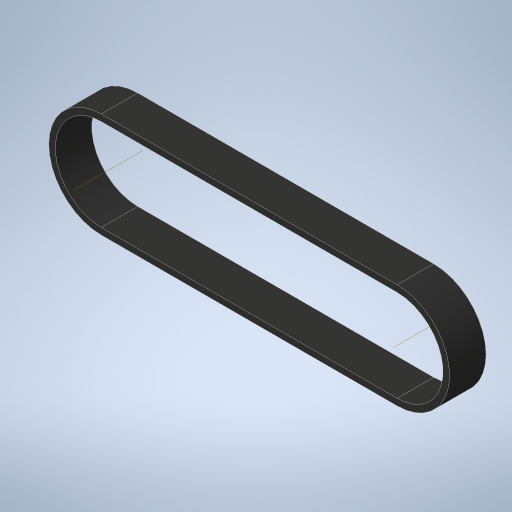
# Autodesk Inventor part: BELT
Saved by Autodesk Inventor 2023.3 (Build 273359000, 359)
## iProperties
RuleStatus: InUse
Created: 2019-01-18
Part Number: BELT
Material: Rubber
Document SubType Name: Modeling
Designer: pctech
Density: 0.93 g/cm^3
Appearance: Rubber - Black
AfterDocOpen0: show
AfterDocNew0: show
Author: pctech
Autodesk Inventor part; units mm, degrees
ref_plane "YZ Plane" through (0, 0, 0) normal (1, 0, 0) x (0, 1, 0)
ref_plane "XZ Plane" through (0, 0, 0) normal (0, 1, 0) x (-1, 0, 0)
ref_plane "XY Plane" through (0, 0, 0) normal (0, 0, 1) x (1, 0, 0)
sketch "Sketch1" plane through (0, 0, 0) normal (0, 0, 1) x (1, 0, 0)
  arc A0 (0, -11.4595) -> (0, 11.4595) centre (0, 0) ccw construction
  arc A1 (-68.9989, 11.4595) -> (-68.9989, -11.4595) centre (-68.9989, 0) ccw construction
  line L0 (0, -11.4595) -> (-68.9989, -11.4595) construction
  line L1 (0, 11.4595) -> (-68.9989, 11.4595) construction
  dimension "Belt_Teeth" = 70
  dimension "Belt_Pitch2" = 3
  dimension "d0" = 22.919
  dimension "d1" = 22.919
  dimension "d2" = 36.0011
  dimension "d3" = 36.0011
  dimension "Center_Distance" = 68.9989
  dimension "d5" = 68.9989
  constraints: 4 end point, 4 point on circle, 4 tangent, 2 centre point, 1 coincident, 1 horizontal alignment
  measures "d0" diameter of A0
  measures "d1" diameter of A1
  measures "Center_Distance" distance of A1.centre point (0, 0)
  measures "d5" distance of L1.start L1.end
sketch "Sketch2" plane through (0, 0, 0) normal (0, 0, 1) x (1, 0, 0)
  line L0 (35.7235, 34.2567) -> (38.7235, 34.2567)
  point P0 (0, 0)
  dimension "Belt_Pitch2" = 3
  constraints: 2 end point, 1 horizontal
  measures "Belt_Pitch2" distance of L0.start L0.end
sketch "Sketch4" plane through (0, 0, 0) normal (0, 0, 1) x (1, 0, 0)
  line L0 (-16.1422, -21.869) -> (-14.1422, -21.869)
  line L1 (-16.1422, -21.869) -> (-16.1422, -20.349)
  arc A0 (-15.5872, -20.904) -> (-16.1422, -20.349) centre (-16.1422, -20.904) ccw
  line L2 (-15.5872, -20.904) -> (-15.5872, -20.959)
  arc A1 (-15.5872, -20.959) -> (-15.4372, -21.109) centre (-15.4372, -20.959) ccw
  line L3 (-15.4372, -21.109) -> (-14.8472, -21.109)
  line L4 (-14.1422, -21.869) -> (-14.1422, -20.349)
  arc A2 (-14.1422, -20.349) -> (-14.6972, -20.904) centre (-14.1422, -20.904) ccw
  arc A3 (-14.8472, -21.109) -> (-14.6972, -20.959) centre (-14.8472, -20.959) ccw
  line L5 (-14.6972, -20.959) -> (-14.6972, -20.904)
  line L6 (0, 11.4595) -> (-68.9989, 11.4595) construction
  arc A4 (-68.9989, 11.4595) -> (-68.9989, -11.4595) centre (-68.9989, 0) ccw construction
  line L7 (0, -11.4595) -> (-68.9989, -11.4595) construction
  arc A5 (0, -11.4595) -> (0, 11.4595) centre (0, 0) ccw construction
  arc A6 (-68.9989, 12.2195) -> (-68.9989, -12.2195) centre (-68.9989, 0) ccw
  line L8 (-68.9989, 12.2195) -> (0, 12.2195)
  arc A7 (0, -12.2195) -> (0, 12.2195) centre (0, 0) ccw
  line L9 (0, -12.2195) -> (-68.9989, -12.2195)
  arc A8 (-68.9989, 10.6995) -> (-68.9989, -10.6995) centre (-68.9989, 0) ccw
  line L10 (-68.9989, 10.6995) -> (0, 10.6995)
  arc A9 (0, -10.6995) -> (0, 10.6995) centre (0, 0) ccw
  line L11 (0, -10.6995) -> (-68.9989, -10.6995)
  point P0 (-15.1422, -21.109)
  point P1 (-15.1422, -21.869)
  dimension "d9" = 2
  dimension "d10" = 1.52
  dimension "d11" = 0.76
  dimension "d12" = 0.555
  dimension "d13" = 0.555
  dimension "d14" = 0.15
  dimension "d15" = 0.15
  dimension "belt_thickness" = 1.52
  dimension "d44" = 0.76
  constraints: 20 end point, 16 point on circle, 8 centre point, 6 tangent, 3 vertical, 2 horizontal, 2 midpoint, 2 point on line, 1 horizontal alignment, 1 vertical alignment, 6 other
  measures "d9" distance of L0.start L0.end
  measures "d10" distance of L0.start L1.end
  measures "d11" distance between parallel lines of L0 L3
  measures "d12" radius of A0
  measures "d13" radius of A2
  measures "d14" radius of A1
  measures "d15" radius of A3
  measures "belt_thickness" radial gap between concentric circles of A6 A8
  measures "d44" radial gap between concentric circles of A4 A6
extrude "Extrusion2" add sketch "Sketch4" along normal mid plane 8.5 contours L8 A7 L9 A6
sketch "Sketch5" plane through (0, 0, 4.25) normal (0, 0, 1) x (1, 0, 0)
  line L0 (-68.9989, 10.6995) -> (0, 10.6995) construction
  arc A0 (0, -10.6995) -> (0, 10.6995) centre (0, 0) ccw construction
  line L1 (0, -10.6995) -> (-68.9989, -10.6995) construction
  arc A1 (-68.9989, 10.6995) -> (-68.9989, -10.6995) centre (-68.9989, 0) ccw construction
  arc A2 (-68.9989, 12.2195) -> (-68.9989, -12.2195) centre (-68.9989, 0) ccw construction
  line L2 (-68.9989, -12.2195) -> (0, -12.2195) construction
  arc A3 (0, -12.2195) -> (0, 12.2195) centre (0, 0) ccw construction
  line L3 (0, 12.2195) -> (-68.9989, 12.2195) construction
  line L4 (-7.7556, -2.6989) -> (-5.7556, -2.6989)
  line L5 (-7.7556, -2.6989) -> (-7.7556, -1.1789) construction
  arc A4 (-7.2006, -1.7339) -> (-7.7556, -1.1789) centre (-7.7556, -1.7339) ccw
  line L6 (-7.2006, -1.7339) -> (-7.2006, -1.7889)
  arc A5 (-7.2006, -1.7889) -> (-7.0506, -1.9389) centre (-7.0506, -1.7889) ccw
  line L7 (-7.0506, -1.9389) -> (-6.4606, -1.9389)
  line L8 (-5.7556, -2.6989) -> (-5.7556, -1.1789)
  arc A6 (-5.7556, -1.1789) -> (-6.3106, -1.7339) centre (-5.7556, -1.7339) ccw
  arc A7 (-6.4606, -1.9389) -> (-6.3106, -1.7889) centre (-6.4606, -1.7889) ccw
  line L9 (-6.3106, -1.7889) -> (-6.3106, -1.7339)
  line L10 (-8.3106, -1.7339) -> (-8.3106, -1.7889)
  arc A8 (-7.7556, -1.1789) -> (-8.3106, -1.7339) centre (-7.7556, -1.7339) ccw
  arc A9 (-8.4606, -1.9389) -> (-8.3106, -1.7889) centre (-8.4606, -1.7889) ccw
  line L11 (-8.4606, -1.9389) -> (-9.0506, -1.9389)
  line L12 (-7.7556, -2.6989) -> (-9.7556, -2.6989)
  line L13 (-9.2006, -1.7889) -> (-9.2006, -1.7339)
  arc A10 (-9.2006, -1.7339) -> (-9.7556, -1.1789) centre (-9.7556, -1.7339) ccw
  line L14 (-9.7556, -2.6989) -> (-9.7556, -1.1789)
  arc A11 (-9.2006, -1.7889) -> (-9.0506, -1.9389) centre (-9.0506, -1.7889) ccw
  line L15 (-17.66, -0.8495) -> (-14.922, -0.8495) construction
  line L16 (-14.922, -0.8495) -> (-14.922, -2.3671) construction
  line L17 (-14.922, -2.3671) -> (-17.66, -2.3671) construction
  line L18 (-17.66, -2.3671) -> (-17.66, -0.8495) construction
  arc A12 (-15.6383, -1.7102) -> (-16.7483, -1.7102) centre (-16.1933, -1.7102) ccw construction
  line L19 (-16.7483, -1.7102) -> (-16.7483, -1.7652) construction
  arc A13 (-16.8983, -1.9152) -> (-16.7483, -1.7652) centre (-16.8983, -1.7652) ccw construction
  line L20 (-16.7483, -1.7102) -> (-16.7483, -1.9152) construction
  line L21 (-15.6383, -1.7102) -> (-15.6383, -1.9152) construction
  point P0 (-6.7556, -1.9389)
  point P1 (-6.7556, -2.6989)
  point P2 (-8.7556, -2.6989)
  point P3 (-8.7556, -1.9389)
  dimension "d22" = 2
  dimension "d23" = 1.52
  dimension "d24" = 0.76
  dimension "d25" = 0.555
  dimension "d26" = 0.555
  dimension "d27" = 0.15
  dimension "d28" = 0.15
  dimension "d29" = 0.76
  dimension "d30" = 1
  dimension "d31" = 2
  dimension "d32" = 0.59
  dimension "d34" = 0.555
  dimension "d35" = 0
  dimension "d36" = 0
  dimension "d37" = 0.15
  dimension "d38" = 0.055
  dimension "d39" = 0.055
  dimension "d40" = 0
  dimension "d41" = 0
  dimension "d42" = 0.205
  dimension "d43" = 0.205
  constraints: 36 end point, 20 point on circle, 13 symmetric about line, 10 centre point, 9 tangent, 4 point on line, 2 midpoint, 2 parallel, 1 horizontal, 1 horizontal alignment, 1 perpendicular, 1 vertical alignment, 4 other
  measures "d22" distance of L4.start L4.end
  measures "d23" distance of L4.start L5.end
  measures "d24" distance between parallel lines of L4 L7
  measures "d25" radius of A4
  measures "d26" radius of A6
  measures "d27" radius of A5
  measures "d28" radius of A7
  measures "d29" distance from line of L8.end L7
  measures "d30" distance from line of L5 point (-6.756, -1.939)
  measures "d31" distance of L8.end L5.end
  measures "d32" distance of A7.centre A5.centre
  measures "d34" radius of A12
  measures "d35" vertical distance of L21.start L19.start
  measures "d36" vertical distance of A12.centre L21.start
  measures "d37" radius of A13
  measures "d38" distance of L6.start L6.end
  measures "d39" distance of L19.start L19.end
  measures "d40" horizontal distance of A13.centre A13.start
  measures "d41" vertical distance of A13.start L20.end
  measures "d42" distance of L19.start L20.end
  measures "d43" distance of L21.start L21.end
equation "\"Belt_Teeth\" = 70"
equation "\"d13\" = d12"
equation "\"d15\" = d14"
equation "\"d44\" = 0.5 * belt_thickness"
equation "\"d26\" = d25"
equation "\"d28\" = d27"
equation "\"d30\" = 0.5 * d22"
equation "\"d31\" = d22"
equation "\"d43\" = d42"
equation "\"Belt_Pitch\" = 3"
equation "\"HTD_5mm\" = 5"
equation "\"GT2_3mm\" = 3"
equation "\"Center_Distance_Copy\" = Center_Distance"
body "Solid2"
